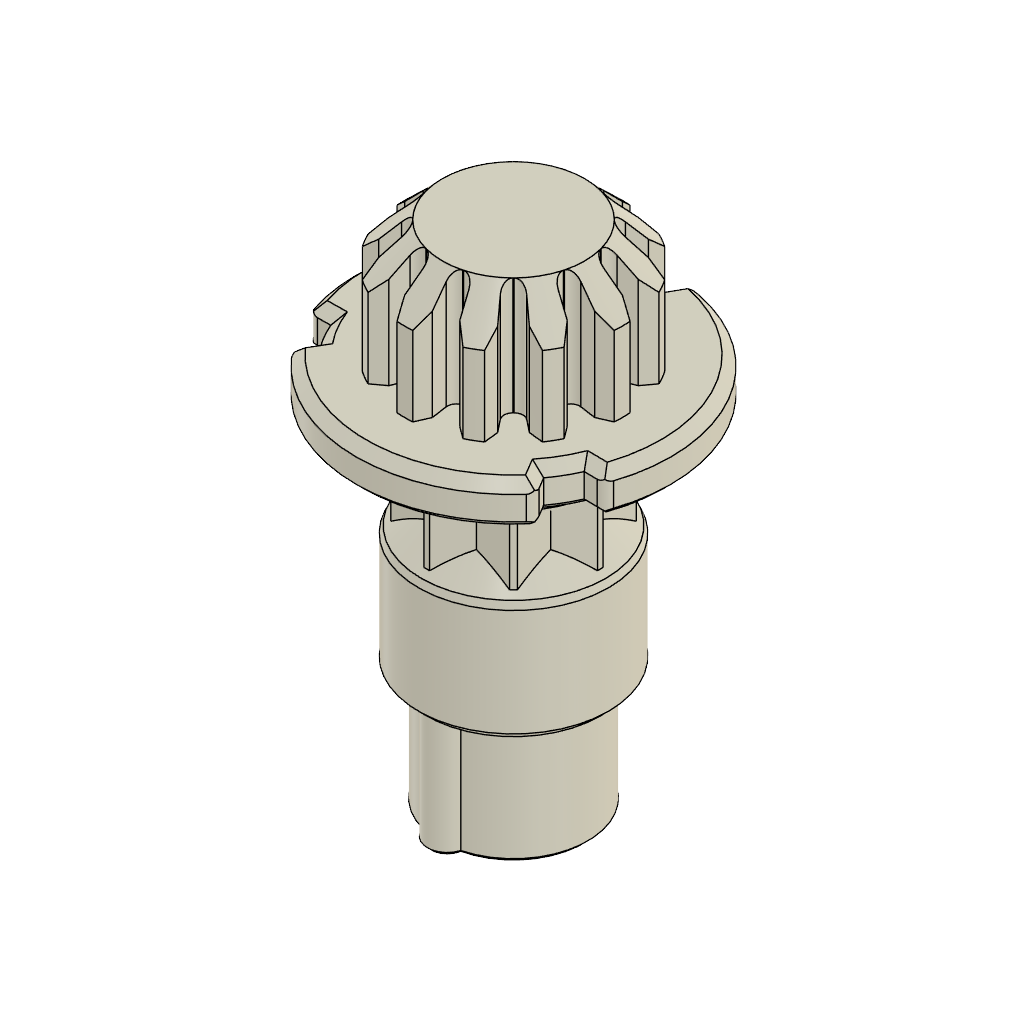
Bit (Low) (Autodesk Fusion 360 design; units mm, degrees)
Autodesk Fusion 360 part; units mm, degrees
sketch "Sketch1" plane through (0, 0, 0) normal (0, 0, 1) x (1, 0, 0)
  circle A0 centre (0, 0) radius 4.35
  line L0 (0, -4.35) -> (0, 4.35) construction
  circle A1 centre (0, 3.35) radius 1
  circle A2 centre (0, -3.35) radius 1
  circle A3 centre (0, 0) radius 3.75
  dimension "d1" = 8.7
  dimension "d8" = 2
  dimension "d10" = 360
  dimension "d11" = 7.5
  constraint coincident A0.centre A3.centre
  constraint coincident A0 L0.start
  constraint coincident A0 L0.end
  constraint vertical L0
  constraint coincident L0 A1.centre
  constraint coincident L0.end A1
  measures "d1" diameter of A0
  measures "d8" diameter of A1
  measures "d11" diameter of A3
extrude "Extrude1" add sketch "Sketch1" along normal blind 6 contours A1 A3 | A2 A3 | A1 A2 A3 | A1 A3 | A2 A3 makes body 1
sketch "Sketch2" plane through (0, 0, 6) normal (0, 0, 1) x (-1, 0, 0)
  circle A0 centre (0, 0) radius 4.8
  dimension "d7" = 9.6
  constraint coincident A0.centre origin
  measures "d7" diameter of A0
extrude "Extrude2" add sketch "Sketch2" along normal blind 6 bodies 1
sketch "Sketch3" plane through (0, 0, 12) normal (0, 0, 1) x (-1, 0, 0)
  circle A0 centre (0, 0) radius 4.8
  line L0 (3.2, -3.2) -> (3.2, 3.2)
  line L1 (3.2, 3.2) -> (-3.2, 3.2)
  line L2 (-3.2, 3.2) -> (-3.2, -3.2)
  line L3 (-3.2, -3.2) -> (3.2, -3.2)
  line L4 (-4.5255, 0) -> (0, -4.5255)
  line L5 (0, 4.5255) -> (-4.5255, 0)
  line L6 (4.5255, 0) -> (0, 4.5255)
  line L7 (0, -4.5255) -> (4.5255, 0)
  dimension "d14" = 6.4
  dimension "d16" = 45
  constraint coincident A0.centre origin
  measures "d14" distance of L1.end L2.end
extrude "Extrude3" add sketch "Sketch3" along normal blind 3.7 contours L0 L3 L7 | L0 L1 L2 L3 L4 L5 L6 L7 | L0 L6 L7 | L3 L4 L7 | L0 L1 L6 | L2 L3 L4 | L1 L5 L6 | L2 L4 L5 | L1 L2 L5 bodies 1
sketch "Sketch4" plane through (0, 0, 0) normal (0, 1, 0) x (1, 0, 0)
  line L0 (-4.8, -12) -> (4.8, -12)
  line L1 (4.8, -12) -> (3.4635, -13.3365)
  line L2 (4.8, -12) -> (4.8, -14.1156) construction
  line L3 (3.4635, -13.3365) -> (0, -13.3365)
  line L4 (0, -13.3365) -> (0, -12)
  dimension "d19" = 45
  dimension "d21" = 3.4635
  constraint coincident L0.end L1.start
  constraint perpendicular L0 L2
  constraint midpoint L0 L4.end
  constraint perpendicular L0 L4
  constraint perpendicular L3 L4
  measures "d19" angle of L1 L2
  measures "d21" distance of L1.end L3.end
revolve "Revolve1" add sketch "Sketch4" angle 360 about axis through (0, 0, 1.75) along (0, 0, 1) bodies 1
chamfer "Chamfer7" distance 0.2 angle 45 13 edges at (0, -4.5255, 13.9873) (3.2, -3.2, 13.9873) (4.5255, 0, 13.9873) (3.2, 3.2, 13.9873) (0, 4.5255, 13.9873) (-3.2, 3.2, 13.9873) (-4.5255, 0, 13.9873) (-3.2, -3.2, 13.9873) (4.4752, 1.7358, 12) (-3.75, 0, 0) (0, 4.35, 0) (3.75, 0, 0) (0, -4.35, 0) on bodies 1
chamfer "Chamfer7" distance 0.4 angle 45 1 edges at (4.4752, 1.7358, 6) on bodies 1
sketch "Sketch16" plane through (0, 0, 15.7) normal (0, 0, 1) x (-1, 0, 0)
  circle A0 centre (0, 0) radius 3.25
  dimension "d84" = 6.5
  constraint coincident A0.centre origin
  measures "d84" diameter of A0
extrude "Extrude12" add sketch "Sketch16" along normal blind 1.5 bodies 1
sketch "Sketch17" plane through (0, 0, 17.2) normal (0, 0, 1) x (-1, 0, 0)
  circle A0 centre (0, 0) radius 3.25
  line L0 (-2.4681, -2.4681) -> (2.4681, -2.4681)
  line L1 (2.4681, -2.4681) -> (2.4681, 2.4681)
  line L2 (2.4681, 2.4681) -> (-2.4681, 2.4681)
  line L3 (-2.4681, 2.4681) -> (-2.4681, -2.4681)
  line L4 (-2.4681, -2.4681) -> (2.4681, 2.4681) construction
  line L5 (2.4681, -2.4681) -> (-2.4681, 2.4681) construction
  line L6 (-2.1145, -2.4681) -> (-2.4681, -2.1145) construction
  dimension "d88" = 0.5
  constraint horizontal L0
  constraint perpendicular L0 L1
  constraint parallel L0 L2
  constraint parallel L1 L3
  constraint coincident L4 A0.centre
  constraint coincident L5 A0.centre
  constraint coincident A0.centre origin
  constraint equal L0 L1
  constraint coincident L0 L6.start
  constraint coincident A0 L6.start
  constraint coincident L3 L6.end
  constraint coincident A0 L6.end
  measures "d88" distance of L6.start L6.end
extrude "Extrude13" add sketch "Sketch17" along normal blind 3.5 contours A0 L0 L1 L2 L3 bodies 1
ref_plane "WorkPlane2" through (0, 0, 15.8) normal (0, 0, 1) x (1, 0, 0)
sketch "Sketch5" plane through (0, 0, 15.8) normal (0, 0, 1) x (-1, 0, 0)
  circle A0 centre (0, 0) radius 4.65
extrude "Extrude4" add sketch "Sketch5" along normal blind 1.8 separate body makes body 2
sketch "Sketch6" plane through (0, 0, 17.6) normal (0, 0, 1) x (-1, 0, 0)
  circle A0 centre (0, 0) radius 4.65
  circle A1 centre (0, 0) radius 7.95
  circle A2 centre (0, 0) radius 7
  line L0 (1.25, -7.8511) -> (0.75, -6.9597)
  line L1 (-0.75, -6.9597) -> (-1.25, -7.8511)
  line L2 (0, -7) -> (0, -7.95) construction
  line L3 (6.4023, 2.8303) -> (7.4243, 2.843)
  line L4 (6.1743, 5.0081) -> (5.6523, 4.1294)
  line L5 (-5.6523, 4.1294) -> (-6.1743, 5.0081)
  line L6 (-7.4243, 2.843) -> (-6.4023, 2.8303)
  line L7 (-0.75, -6.9597) -> (0.75, -6.9597) construction
  line L8 (-1.25, -7.8511) -> (1.25, -7.8511) construction
  dimension "d24" = 15.9
  dimension "d109" = 14
  dimension "d113" = 360
  dimension "d137" = 2.5
  dimension "d138" = 1.5
  constraint coincident A0.centre A1.centre
  constraint coincident A1 L0.start
  constraint coincident A2 L0.end
  constraint coincident A2 L1.start
  constraint coincident A1 L1.end
  constraint coincident A2 L2.start
  constraint coincident A1 L2.end
  constraint vertical L2
  constraint symmetric L0 L1 L2
  constraint perpendicular L2 L7
  measures "d24" diameter of A1
  measures "d109" diameter of A2
  measures "d137" distance of L0.start L1.end
  measures "d138" distance of L0.end L1.start
extrude "Extrude5" add sketch "Sketch6" along normal blind 2 contours A0 | A1 A2 L0 L3 | A1 A2 L4 L5 | A2 | A1 A2 L1 L6 bodies 2
hole "Hole1" at (0, 0, 0) direction (0, 0, 1) diameter 4.7 depth 12.8 tip angle 180 bodies 1 2
chamfer "Chamfer1" distance 0.5 angle 45 12 edges at (6.8849, 3.975, 19.6) (-1, 7.4054, 19.6) (0, 7, 19.6) (1, 7.4054, 19.6) (-6.8849, 3.975, 19.6) (6.9133, -2.8367, 19.6) (6.0622, -3.5, 19.6) (5.9133, -4.5687, 19.6) (0, -7.95, 19.6) (-6.9133, -2.8367, 19.6) (-6.0622, -3.5, 19.6) (-5.9133, -4.5687, 19.6) on bodies 1 2
chamfer "Chamfer1" distance 0.3 angle 45 12 edges at (0, -7.95, 17.6) (-5.9133, -4.5687, 17.6) (-6.0622, -3.5, 17.6) (-6.9133, -2.8367, 17.6) (-6.8849, 3.975, 17.6) (-1, 7.4054, 17.6) (0, 7, 17.6) (1, 7.4054, 17.6) (6.8849, 3.975, 17.6) (6.9133, -2.8367, 17.6) (6.0622, -3.5, 17.6) (5.9133, -4.5687, 17.6) on bodies 1 2
chamfer "Chamfer1" distance 0.2 angle 45 1 edges at (2.191, 0.8498, 0) on bodies 1 2
sketch "Sketch20" plane through (0, 0, 19.6) normal (0, 0, 1) x (-1, 0, 0)
  arc A0 (6.0695, 2.3262) -> (5.0493, 4.0933) centre (0, 0) ccw
  line L0 (5.0493, 4.0933) -> (5.562, 4.9564)
  arc A1 (5.562, 4.9564) -> (-5.562, 4.9564) centre (0, 0) ccw
  line L1 (-5.562, 4.9564) -> (-5.0493, 4.0933)
  arc A2 (-5.0493, 4.0933) -> (-6.0695, 2.3262) centre (0, 0) ccw
  line L2 (-6.0695, 2.3262) -> (-7.0734, 2.3386)
  arc A3 (-7.0734, 2.3386) -> (-1.5114, -7.2951) centre (0, 0) ccw
  line L3 (-1.5114, -7.2951) -> (-1.0202, -6.4194)
  arc A4 (-1.0202, -6.4194) -> (1.0202, -6.4194) centre (0, 0) ccw
  line L4 (1.0202, -6.4194) -> (1.5114, -7.2951)
  arc A5 (1.5114, -7.2951) -> (7.0734, 2.3386) centre (0, 0) ccw
  line L5 (7.0734, 2.3386) -> (6.0695, 2.3262)
  circle A6 centre (0, 0) radius 3.6
  dimension "d140" = 7.2
  measures "d140" diameter of A6
extrude "Extrude16" add sketch "Sketch20" along normal blind 5.9 contours A6 bodies 2
sketch "Sketch21" plane through (0, 0, 19.6) normal (0, 0, 1) x (-1, 0, 0)
  circle A0 centre (0, 0) radius 3.6
  line L0 (0, 0) -> (0, -0.2226)
  line L1 (0, -0.2226) -> (0, -3.6) construction
  line L2 (0, 0) -> (0.7, -4.7992)
  line L3 (0, 0) -> (-0.7, -4.7992)
  circle A1 centre (0, 0) radius 5.5
  line L4 (0.7, -4.7992) -> (0.4, -5.4854)
  line L5 (-0.7, -4.7992) -> (-0.4, -5.4854)
  dimension "d141" = 7.2
  dimension "d142" = 4.85
  dimension "d143" = 1.4
  dimension "d144" = 11
  dimension "d145" = 0.8
  constraint coincident A0.centre L0.start
  constraint vertical L0
  constraint coincident A0 L1.end
  constraint parallel L0 L1
  constraint symmetric L1 A0.centre L0.start
  constraint symmetric L1 L2.end L3.end
  constraint concentric A0 A1
  constraint coincident A1 L4.end
  constraint coincident A1 L5.end
  constraint symmetric L1 L4 L5
  measures "d141" diameter of A0
  measures "d142" distance of A0.centre L2.end
  measures "d143" distance of L2.end L3.end
  measures "d144" diameter of A1
  measures "d145" distance of L4.end L5.end
extrude "Extrude17" add sketch "Sketch21" along normal up to surface (5.9 mm away) contours A0 L2 L3 A1 L4 L5 picked at (-0.0579, -4.3981) bodies 2
fillet "Fillet5" radius 0.45 2 edges at (-0.5196, 3.5623, 22.55) (0.5196, 3.5623, 22.55) on bodies 2
pattern_circular "C-Pattern2" count 12 over 360 about axis through (0, 0, 1.75) along (0, 0, 1) of "Extrude17", "Fillet5"
chamfer "Chamfer9" distance 1.9 angle 45 12 edges at (-2.75, -4.7631, 25.5) (-4.7631, -2.75, 25.5) (-5.5, 0, 25.5) (-4.7631, 2.75, 25.5) (-2.75, 4.7631, 25.5) (0, 5.5, 25.5) (0, -5.5, 25.5) (2.75, 4.7631, 25.5) (4.7631, 2.75, 25.5) (5.5, 0, 25.5) (4.7631, -2.75, 25.5) (2.75, -4.7631, 25.5) on bodies 2
sketch "Sketch18" plane through (0, 0, 15.8) normal (0, 0, -1) x (1, 0, 0)
  circle A0 centre (0, 0) radius 3.25 construction
  circle A1 centre (0, 0) radius 3.35
  dimension "d92" = 0.1
extrude "Extrude14" cut sketch "Sketch18" against normal blind 1.5 bodies 2
sketch "Sketch19" plane through (0, 0, 17.3) normal (0, 0, -1) x (1, 0, 0)
  arc A0 (2.4681, 2.1145) -> (2.1145, 2.4681) centre (0, 0) ccw construction
  line L0 (2.4681, 2.1145) -> (2.4681, -2.1145) construction
  arc A1 (2.1145, -2.4681) -> (2.4681, -2.1145) centre (0, 0) ccw construction
  line L1 (2.1145, -2.4681) -> (-2.1145, -2.4681) construction
  arc A2 (-2.4681, -2.1145) -> (-2.1145, -2.4681) centre (0, 0) ccw construction
  line L2 (-2.4681, -2.1145) -> (-2.4681, 2.1145) construction
  arc A3 (-2.1145, 2.4681) -> (-2.4681, 2.1145) centre (0, 0) ccw construction
  line L3 (-2.1145, 2.4681) -> (2.1145, 2.4681) construction
  arc A4 (-2.5681, -2.1512) -> (-2.1512, -2.5681) centre (0, 0) ccw
  line L4 (2.1512, -2.5681) -> (-2.1512, -2.5681)
  arc A5 (2.1512, -2.5681) -> (2.5681, -2.1512) centre (0, 0) ccw
  line L5 (2.5681, 2.1512) -> (2.5681, -2.1512)
  arc A6 (2.5681, 2.1512) -> (2.1512, 2.5681) centre (0, 0) ccw
  line L6 (-2.1512, 2.5681) -> (2.1512, 2.5681)
  arc A7 (-2.1512, 2.5681) -> (-2.5681, 2.1512) centre (0, 0) ccw
  line L7 (-2.5681, -2.1512) -> (-2.5681, 2.1512)
  dimension "d95" = -0.1
extrude "Extrude15" cut sketch "Sketch19" against normal blind 3.5 bodies 2
fillet "Fillet1" radius 0.25 2 edges at (4.3353, 1.6815, 15.8) (4.3353, 1.6815, 17.6) on bodies 2
fillet "Fillet1" radius 0.5 6 edges at (7.4243, -2.843, 18.5) (6.1743, -5.0081, 18.5) (1.25, 7.8511, 18.5) (-1.25, 7.8511, 18.5) (-7.4243, -2.843, 18.5) (-6.1743, -5.0081, 18.5) on bodies 2
hole "Hole3" at (0, 0, 12.8) direction (0, 0, 1) diameter 2 depth 10 tip angle 180 counterbore diameter 4 counterbore depth 2 bodies 1 2
equation "d12 = 11.9 mm - 5.9 mm"
equation "d17 = 15.6 mm - 11.9 mm"
equation "d21 = ( 6.927 / 2 ) * 1 mm"
equation "d22 = 17.4 mm - 15.6 mm"
